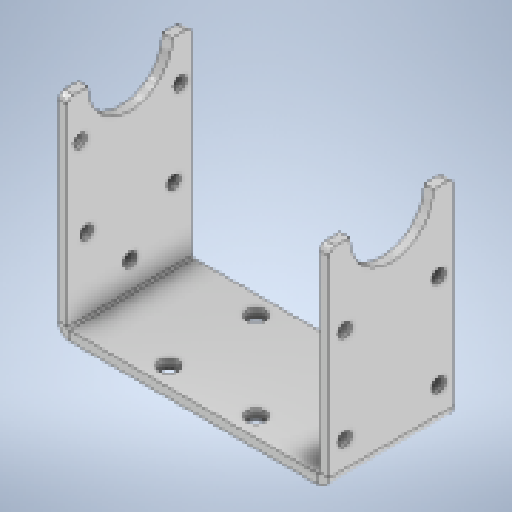
# Autodesk Inventor part: axis_10_top_frame
Saved by Autodesk Inventor 2026.1 (Build 301233000, 233)
## iProperties
Created: 2025-05-04
Part Number: axis_10_top_frame
Material: Aluminum 6061-AHC
Document SubType Name: Sheet Metal
Designer: User
Density: 2.7 g/cm^3
Sheet Metal Rule: Default_mm
Appearance: Aluminum - Dark
Flat Pattern Width: 2 cm
Flat Pattern Length: 10.5259 cm
Flat Pattern Area: 21.0517 cm^2
Sheet Metal Width: 20.000 mm
Sheet Metal Length: 105.259 mm
Sheet Metal Area: 2105.171 mm^2
Author: User
Autodesk Inventor part; units mm, degrees
ref_plane "YZ Plane" through (0, 0, 0) normal (1, 0, 0) x (0, 1, 0)
ref_plane "XZ Plane" through (0, 0, 0) normal (0, 1, 0) x (-1, 0, 0)
ref_plane "XY Plane" through (0, 0, 0) normal (0, 0, 1) x (1, 0, 0)
sketch "Sketch1" plane through (0, 0, 0) normal (0, 1, 0) x (-1, 0, 0)
  line L0 (20.25, -10) -> (-20.25, -10)
  line L1 (-20.25, -10) -> (-20.25, 10)
  line L2 (-20.25, 10) -> (20.25, 10)
  line L3 (20.25, 10) -> (20.25, -10)
  point P0 (0, 0)
  dimension "d0" = 40.5
  dimension "d1" = 20
  dimension "d2" = 10
  dimension "d3" = 20.25
  measures "d0" distance of L0.start L0.end
  measures "d1" distance of L2.end L0.start
  measures "d2" distance from line of L0 point (0, 0)
  measures "d3" distance from line of point (0, 0) L3
extrude "Plate1" add sketch "Sketch1" along normal blind 1.5
sketch "Sketch2" plane through (21.75, 0, -10) normal (-1, 0, 0) x (0, -1, 0)
  line L0 (0, 20) -> (0, 0)
  line L1 (0, 0) -> (-43.5, 0)
  line L2 (-43.5, 0) -> (-43.5, 20)
  line L3 (-43.5, 20) -> (0, 20)
  constraints: 8 end point
edge flange "Flange1" height 43.5 angle 90 thickness 1.5 bend radius 0.31 thickness toward (-1, 0, 0) relief tear relief width 1.5 relief depth 0.75 edges at (20.25, 1.5, 0) wall of the first edge with corners at (21.75, 0, 10) (21.75, 0, -10) (21.75, 43.5, -10) (21.75, 43.5, 10)
bend "Bend1"
corner "Corner1"
sketch "Sketch3" plane through (-21.75, 0, 10) normal (1, 0, 0) x (0, 1, 0)
  line L0 (0, -20) -> (0, 0)
  line L1 (0, 0) -> (43.5, 0)
  line L2 (43.5, 0) -> (43.5, -20)
  line L3 (43.5, -20) -> (0, -20)
  constraints: 8 end point
edge flange "Flange2" height 43.5 angle 90 thickness 1.5 bend radius 0.31 thickness toward (1, 0, 0) relief tear relief width 1.5 relief depth 0.75 edges at (-20.25, 1.5, 0) wall of the first edge with corners at (-21.75, 0, -10) (-21.75, 0, 10) (-21.75, 43.5, 10) (-21.75, 43.5, -10)
bend "Bend2"
corner "Corner2"
sketch "Sketch4" plane through (21.75, 43.5, 10) normal (1, 0, 0) x (0, 0, -1)
  circle A0 centre (10, -9.9) radius 6.75
  line L0 (0, 0) -> (20, 0) projected
  line L1 (20, 0) -> (20, -41.69) projected
  point P0 (10, -43.5)
  dimension "d25" = 9.9
  dimension "d26" = 13.5
  dimension "d27" = 10
  constraints: 1 centre point
  measures "d25" distance from line of A0.centre L0
  measures "d26" diameter of A0
  measures "d27" distance from line of L1 A0.centre
extrude "Extrusion1" cut sketch "Sketch4" against normal blind 50
sketch "Sketch5" plane through (21.75, 43.5, 10) normal (1, 0, 0) x (0, 0, -1)
  circle A0 centre (10, -9.9) radius 6.75 projected
  line L0 (0, 0) -> (20, 0) projected
  line L1 (-4, 0) -> (24, 0)
  line L2 (24, 0) -> (24, -9.9)
  line L3 (24, -9.9) -> (-4, -9.9)
  line L4 (-4, -9.9) -> (-4, 0)
  line L5 (0, -41.69) -> (0, 0) projected
  point P0 (10, -43.5)
  point P1 (20, 0)
  dimension "d30" = 9.9
  dimension "d31" = 28
  dimension "d32" = 4
  constraints: 8 end point, 2 parallel, 1 horizontal, 1 perpendicular, 1 point on line
  measures "d30" distance of L3.end L1.start
  measures "d31" distance of L1.start L1.end
  measures "d32" distance between parallel lines of L5 L4
extrude "Extrusion2" cut sketch "Sketch5" against normal blind 50 contours L3 A0 | A0 L3 L5 L0 L1 L2 | L3 L4 L1 L5 picked at (11.6841, -8.408)
fillet "Fillet1" radius 1 4 edges at (-21, 33.6, 10) (-21, 33.6, -10) (21, 33.6, -10) (21, 33.6, 10)
sketch "Sketch11" plane through (0, 1.5, 0) normal (0, 1, 0) x (1, 0, 0)
  circle A0 centre (7, 7) radius 1.5
  line L0 (-19.94, 10) -> (19.94, 10) projected
  line L1 (-19.94, 10) -> (-19.94, -10) projected
  circle A1 centre (-7, 7) radius 1.5
  circle A2 centre (7, -7) radius 1.5
  circle A3 centre (-7, -7) radius 1.5
  point P0 (0, 0)
  dimension "d71" = 7
  dimension "d72" = 3
  dimension "d73" = 7
  dimension "d76" = 14
  dimension "d79" = 14
  constraints: 4 centre point, 1 horizontal, 1 vertical, 6 other
  measures "d71" horizontal distance of A0.centre point (0, 0)
  measures "d72" diameter of A0
  measures "d73" horizontal distance of A0.centre point (0, 0)
  measures "d76" distance of A0.centre A1.centre
  measures "d79" distance of A0.centre A2.centre
extrude "Extrusion3" cut sketch "Sketch11" against normal through all
sketch "Sketch12" plane through (-21.75, 1.81, -10) normal (-1, 0, 0) x (0, 0, 1)
  circle A0 centre (18, 24.89) radius 0.7835
  circle A1 centre (10, 24.79) radius 0.7835
  circle A2 centre (17, 11.67) radius 0.7835
  circle A3 centre (3, 11.67) radius 0.7835
  circle A4 centre (10, 4.37) radius 0.7835
  circle A5 centre (2, 24.89) radius 0.7835
  point P0 (10, -1.81)
  constraints: 6 centre point, 12 other
hole "Hole6" at (-21.75, 26.7, -8) at (-21.75, 26.7, 8) at (-21.75, 13.48, 7) at (-21.75, 6.18, 0) at (-21.75, 13.48, -7) direction (1, 0, 0) diameter 2.1 depth 1.5
sketch "Sketch13" plane through (21.75, 1.81, 10) normal (1, 0, 0) x (0, 0, -1)
  circle A0 centre (17.525, 4.19) radius 0.7835
  circle A1 centre (2.475, 4.19) radius 0.7835
  circle A2 centre (2.475, 19.29) radius 0.7835
  circle A3 centre (17.525, 19.29) radius 0.7835
  point P0 (10, -1.81)
  constraints: 4 centre point, 8 other
hole "Hole7" at (21.75, 21.1, 7.525) at (21.75, 21.1, -7.525) at (21.75, 6, -7.525) at (21.75, 6, 7.525) direction (-1, 0, 0) diameter 2.1 depth 1.5
equation "\"d89\" = Thickness"
equation "\"d96\" = Thickness"
equation "\"d4\" = Thickness"
equation "\"d5\" = BendReliefWidth"
equation "\"d6\" = BendReliefDepth"
equation "\"d7\" = MinimumRemnant"
equation "\"d8\" = TransitionRadius"
equation "\"d11\" = BendRadius"
equation "\"d12\" = CornerReliefSize"
equation "\"d13\" = GapSize"
equation "\"d14\" = JacobiRadiusSize"
equation "\"d15\" = BendReliefWidth"
equation "\"d16\" = BendReliefDepth"
equation "\"d17\" = MinimumRemnant"
equation "\"d18\" = TransitionRadius"
equation "\"d21\" = BendRadius"
equation "\"d22\" = CornerReliefSize"
equation "\"d23\" = GapSize"
equation "\"d24\" = JacobiRadiusSize"
equation "\"BendReliefWidth\" = Thickness"
equation "\"BendReliefDepth\" = 0.5 * Thickness"
equation "\"CornerReliefSize\" = 4 * Thickness"
equation "\"MinimumRemnant\" = 2 * Thickness"
equation "\"TransitionRadius\" = BendRadius"
equation "\"JacobiRadiusSize\" = BendRadius"
equation "\"GapSize\" = Thickness"
equation "\"Thickness\" = 1.5"
equation "\"BendRadius\" = 0.31"
body "Solid1"
